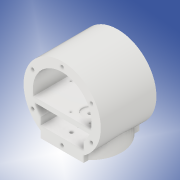
# Autodesk Inventor part: SJ003
Saved by Autodesk Inventor 2017 (Build 210142000, 142)
## iProperties
Created: 2017-06-01
Part Number: SJ003
Material: ABS Plastic
Document SubType Name: Modeling
Designer: Zach
Density: 1.06 g/cm^3
Appearance: CR White
Author: Zach
Autodesk Inventor part; units mm, degrees
ref_plane "YZ Plane" through (0, 0, 0) normal (1, 0, 0) x (0, 1, 0)
ref_plane "XZ Plane" through (0, 0, 0) normal (0, 1, 0) x (-1, 0, 0)
ref_plane "XY Plane" through (0, 0, 0) normal (0, 0, 1) x (1, 0, 0)
sketch "Sketch1" plane through (0, 0, 0) normal (0, 0, 1) x (1, 0, 0)
  circle A0 centre (0, 0) radius 62.5
  circle A1 centre (0, 0) radius 47.5
  dimension "d0" = 125
  dimension "d1" = 15
  constraints: 2 centre point, 1 coincident
  measures "d0" diameter of A0
  measures "d1" radial gap between concentric circles of A0 A1
extrude "Extrusion1" add sketch "Sketch1" along normal mid plane 90
sketch "Sketch20" plane through (0, 0, -45) normal (0, 0, -1) x (-1, 0, 0)
  line L0 (34.641, -62.5) -> (-34.641, -62.5)
  line L1 (-34.641, -62.5) -> (-34.641, -32.5)
  line L2 (-34.641, -32.5) -> (34.641, -32.5)
  line L3 (34.641, -32.5) -> (34.641, -62.5)
  circle A0 centre (0, 0) radius 62.5 projected
  circle A1 centre (0, 0) radius 47.5 projected
  point P0 (0, -62.5)
  dimension "d95" = 30
  constraints: 8 end point, 2 point on circle, 1 horizontal, 1 midpoint, 1 parallel, 1 perpendicular, 1 tangent, 1 vertical alignment
  measures "d95" distance of L0.end L1.end
extrude "Extrusion20" add sketch "Sketch20" against normal blind 90 contours L0 A0 L3 | L0 L1 A0 | A0 L1 A1 L3 | A1 L2 picked at (-15.536, -49.9747) picked at (9.1087, -34.6176)
sketch "Sketch30" plane through (-34.641, -62.5, -45) normal (0, -1, 0) x (1, 0, 0)
  circle A0 centre (34.641, 45) radius 50.75 construction
  line L0 (0, 0) -> (0, 90)
  line L1 (69.282, 0) -> (69.282, 90)
  line L2 (0, 0) -> (0, 90)
  arc A1 (0, 82.0886) -> (0, 7.9114) centre (34.641, 45) ccw
  line L3 (69.282, 0) -> (69.282, 90)
  arc A2 (69.282, 7.9114) -> (69.282, 82.0886) centre (34.641, 45) ccw
  line L4 (69.282, 7.9114) -> (69.282, 82.0886)
  line L5 (0, 7.9114) -> (0, 82.0886)
  dimension "d149" = 101.5
  constraints: 12 end point, 8 point on circle, 4 point on line, 3 centre point, 2 concentric, 1 coincident, 1 parallel
  measures "d149" diameter of A0
extrude "Extrusion28" add sketch "Sketch30" against normal blind 30
sketch "Sketch2" plane through (0, 0, 45) normal (0, 0, 1) x (1, 0, 0)
  circle A0 centre (0, 55) radius 2.5
  circle A1 centre (-47.6314, 27.5) radius 2.5
  circle A2 centre (-47.6314, -27.5) radius 2.5
  circle A3 centre (0, -55) radius 2.5
  circle A4 centre (47.6314, -27.5) radius 2.5
  circle A5 centre (47.6314, 27.5) radius 2.5
  point P0 (0, 0)
  dimension "d4" = 5
  dimension "d5" = 55
  dimension "d8" = 360
  constraints: 6 centre point, 13 other
  measures "d4" diameter of A0
  measures "d5" distance of point (0, 0) A0.centre
extrude "Extrusion2" cut sketch "Sketch2" against normal through all
sketch "Sketch21" plane through (-34.641, -62.5, -45) normal (0, -1, 0) x (1, 0, 0)
  line L0 (0, 90) -> (69.282, 90) projected
  line L1 (0, 0) -> (0, 7.9114) projected
  line L2 (0, 0) -> (69.282, 0) projected
  line L3 (69.282, 0) -> (69.282, 7.9114) projected
  circle A0 centre (34.641, 45) radius 30 construction
  circle A1 centre (34.641, 45) radius 18.5
  line L4 (34.641, 45) -> (34.641, 75) construction
  circle A2 centre (34.641, 75) radius 2.5
  circle A3 centre (8.6603, 60) radius 2.5
  circle A4 centre (8.6603, 30) radius 2.5
  circle A5 centre (34.641, 15) radius 2.5
  circle A6 centre (60.6218, 30) radius 2.5
  circle A7 centre (60.6218, 60) radius 2.5
  line L5 (0, 82.0886) -> (0, 90) projected
  arc A8 (0, 82.0886) -> (0, 7.9114) centre (34.641, 45) ccw projected
  arc A9 (69.282, 7.9114) -> (69.282, 82.0886) centre (34.641, 45) ccw projected
  line L6 (69.282, 82.0886) -> (69.282, 90) projected
  dimension "d99" = 60
  dimension "d100" = 37
  dimension "d101" = 5
  dimension "d104" = 360
  constraints: 7 centre point, 3 coincident, 2 end point, 1 vertical, 1 vertical alignment, 15 other
  measures "d100" diameter of A1
  measures "d101" diameter of A2
extrude "Extrusion21" cut sketch "Sketch21" against normal blind 50 contours A1 | A2 | A3 | A4 | A5 | A6 | A7
sketch "Sketch24" plane through (0, 0, 45) normal (0, 0, 1) x (1, 0, 0)
  line L0 (34.641, -32.5) -> (-34.641, -32.5) projected
  line L1 (34.641, -32.5) -> (-34.641, -32.5)
  line L2 (-34.641, -32.5) -> (-34.641, -44.5)
  line L3 (-34.641, -44.5) -> (34.641, -44.5)
  line L4 (34.641, -44.5) -> (34.641, -32.5)
  point P0 (0, 0)
  dimension "d115" = 12
  constraints: 8 end point, 2 parallel, 1 horizontal, 1 perpendicular, 1 vertical alignment
  measures "d115" distance of L2.end L1.end
extrude "Extrusion24" cut sketch "Sketch24" against normal through all
sketch "Sketch25" plane through (0, 0, -45) normal (0, 0, -1) x (-1, 0, 0)
  arc A0 (34.641, -32.5) -> (-34.641, -32.5) centre (0, 0) ccw projected
  line L0 (-46.5403, -9.5) -> (46.5403, -9.5)
  line L1 (46.5403, -9.5) -> (46.5403, -17.5)
  line L2 (46.5403, -17.5) -> (-46.5403, -17.5)
  line L3 (-46.5403, -17.5) -> (-46.5403, -9.5)
  line L4 (34.641, -44.5) -> (-34.641, -44.5) projected
  dimension "d119" = 8
  dimension "d120" = 27
  constraints: 8 end point, 2 parallel, 2 point on circle, 1 horizontal, 1 perpendicular
  measures "d119" distance between parallel lines of L2 L0
  measures "d120" distance between parallel lines of L4 L2
extrude "Extrusion25" add sketch "Sketch25" against normal blind 90 contours L1 L2 A0 | A0 L2 L0 | A0 L2 L3
sketch "Sketch28" plane through (-46.5403, -9.5, -45) normal (0, 1, 0) x (1, 0, 0)
  circle A0 centre (46.5403, -45) radius 18.5 construction
  circle A1 centre (24.9735, -23.4332) radius 12.5 construction
  circle A2 centre (9.4735, -7.9332) radius 1.5
  line L0 (40.4735, -38.9332) -> (9.4735, -38.9332) construction
  line L1 (9.4735, -38.9332) -> (9.4735, -7.9332) construction
  line L2 (9.4735, -7.9332) -> (40.4735, -7.9332) construction
  line L3 (40.4735, -7.9332) -> (40.4735, -38.9332) construction
  line L4 (40.4735, -38.9332) -> (9.4735, -7.9332) construction
  line L5 (9.4735, -38.9332) -> (40.4735, -7.9332) construction
  circle A3 centre (9.4735, -38.9332) radius 1.5
  circle A4 centre (40.4735, -38.9332) radius 1.5
  circle A5 centre (40.4735, -7.9332) radius 1.5
  circle A6 centre (24.9735, -23.4332) radius 3
  circle A7 centre (68.1071, -66.5668) radius 12.5 construction
  circle A8 centre (52.6071, -51.0668) radius 1.5
  line L6 (83.6071, -82.0668) -> (52.6071, -82.0668) construction
  line L7 (52.6071, -82.0668) -> (52.6071, -51.0668) construction
  line L8 (52.6071, -51.0668) -> (83.6071, -51.0668) construction
  line L9 (83.6071, -51.0668) -> (83.6071, -82.0668) construction
  line L10 (83.6071, -82.0668) -> (52.6071, -51.0668) construction
  line L11 (52.6071, -82.0668) -> (83.6071, -51.0668) construction
  circle A9 centre (52.6071, -82.0668) radius 1.5
  circle A10 centre (83.6071, -82.0668) radius 1.5
  circle A11 centre (83.6071, -51.0668) radius 1.5
  circle A12 centre (68.1071, -66.5668) radius 3
  line L12 (46.5403, -45) -> (68.1071, -66.5668) construction
  line L13 (46.5403, -45) -> (46.5403, -141.3744) construction
  line L14 (46.5403, -45) -> (24.9735, -23.4332) construction
  line L15 (46.5403, -45) -> (77.0403, -45) construction
  dimension "d123" = 25
  dimension "d124" = 3
  dimension "d125" = 30.5
  dimension "d126" = 31
  dimension "d127" = 31
  dimension "d128" = 3
  dimension "d129" = 3
  dimension "d130" = 3
  dimension "d131" = 6
  dimension "d132" = 25
  dimension "d133" = 3
  dimension "d134" = 31
  dimension "d135" = 31
  dimension "d136" = 3
  dimension "d137" = 3
  dimension "d138" = 3
  dimension "d139" = 6
  dimension "d140" = 30.5
  dimension "d147" = 45
  dimension "d148" = 135
  constraints: 32 end point, 12 centre point, 12 coincident, 5 midpoint, 4 parallel, 3 horizontal, 2 perpendicular, 1 equal length, 1 vertical
  measures "d123" diameter of A1
  measures "d124" diameter of A2
  measures "d125" distance of point (46.54, -45) A1.centre
  measures "d126" distance of L1.end L2.end
  measures "d127" distance of L0.end L1.end
  measures "d128" diameter of A3
  measures "d129" diameter of A4
  measures "d130" diameter of A5
  measures "d131" diameter of A6
  measures "d132" diameter of A7
  measures "d133" diameter of A8
  measures "d134" distance of L7.end L8.end
  measures "d135" distance of L7.start L7.end
  measures "d136" diameter of A9
  measures "d137" diameter of A10
  measures "d138" diameter of A11
  measures "d139" diameter of A12
  measures "d140" distance of A7.centre point (46.54, -45)
  measures "d147" angle of L13 L12
  measures "d148" angle of L15 L14
extrude "Extrusion26" cut sketch "Sketch28" against normal blind 15
sketch "Sketch29" plane through (-46.5403, -9.5, 45) normal (0, 1, 0) x (1, 0, 0)
  circle A0 centre (68.1071, 23.4332) radius 3 projected
  circle A1 centre (24.9735, 66.5668) radius 3 projected
  circle A2 centre (68.1071, 23.4332) radius 12.5
  circle A3 centre (24.9735, 66.5668) radius 12.5
  point P0 (46.5403, 45)
  dimension "d143" = 25
  dimension "d144" = 25
  constraints: 2 centre point, 2 coincident
  measures "d143" diameter of A2
  measures "d144" diameter of A3
extrude "Extrusion27" cut sketch "Sketch29" against normal blind 2
body "Solid1"
